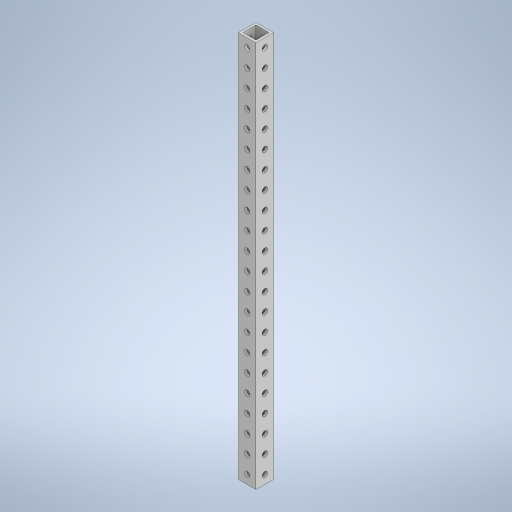
# Autodesk Inventor part: DriveHouseConnector-Length
Saved by Autodesk Inventor 2023 (Build 270158000, 158)
## iProperties
Created: 2022-09-20
Part Number: DriveHouseConnector-Length
Material: Generic
Document SubType Name: Modeling
Designer: seene
Density: 1 g/cm^3
Appearance: Default
Author: seene
Autodesk Inventor part; units mm, degrees
ref_plane "YZ Plane" through (0, 0, 0) normal (1, 0, 0) x (0, 1, 0)
ref_plane "XZ Plane" through (0, 0, 0) normal (0, 1, 0) x (-1, 0, 0)
ref_plane "XY Plane" through (0, 0, 0) normal (0, 0, 1) x (1, 0, 0)
sketch "Sketch1" plane through (0, 0, 0) normal (0, 1, 0) x (-1, 0, 0)
  line L0 (-12.7, 12.7) -> (12.7, 12.7)
  line L1 (12.7, 12.7) -> (12.7, -12.7)
  line L2 (12.7, -12.7) -> (-12.7, -12.7)
  line L3 (-12.7, -12.7) -> (-12.7, 12.7)
  line L4 (-12.7, 12.7) -> (12.7, -12.7) construction
  line L5 (12.7, 12.7) -> (-12.7, -12.7) construction
  line L6 (9.525, -9.525) -> (9.525, 9.525)
  line L7 (9.525, 9.525) -> (-9.525, 9.525)
  line L8 (-9.525, 9.525) -> (-9.525, -9.525)
  line L9 (-9.525, -9.525) -> (9.525, -9.525)
  point P0 (0, 0)
  dimension "d0" = 25.4
  dimension "d1" = 25.4
  dimension "d2" = 3.175
  constraints: 20 end point, 4 parallel, 2 midpoint, 2 perpendicular, 1 horizontal, 3 other
  measures "d0" distance of L1.end L2.end
  measures "d1" distance of L0.end L1.end
  measures "d2" distance between parallel lines of L1 L6
extrude "Extrusion1" add sketch "Sketch1" along normal blind 558.8
sketch "Sketch3" plane through (12.7, 0, 12.7) normal (1, 0, 0) x (0, 0, -1)
  line L0 (0, 0) -> (25.4, 0) projected
  line L1 (0, 0) -> (0, 558.8) projected
  point P0 (12.7, 0)
  point P1 (12.7, 12.7)
  dimension "d5" = 12.7
  dimension "d6" = 12.7
  measures "d5" distance from line of L0 point (12.7, 12.7)
  measures "d6" distance from line of L1 point (12.7, 12.7)
hole "Hole1" at (0, 12.7, 12.7) direction (0, 0, -1) diameter 7.9375 end through all
sketch "Sketch4" plane through (-12.7, 0, 12.7) normal (0, 0, 1) x (1, 0, 0)
  line L0 (0, 0) -> (25.4, 0) projected
  line L1 (25.4, 0) -> (25.4, 558.8) projected
  point P0 (12.7, 0)
  point P1 (12.7, 12.7)
  dimension "d8" = 12.7
  dimension "d10" = 12.7
  measures "d8" distance from line of L0 point (12.7, 12.7)
  measures "d10" distance from line of L1 point (12.7, 12.7)
hole "Hole2" at (12.7, 12.7, 0) direction (-1, 0, 0) diameter 7.9375 end through all
pattern_linear "Rectangular Pattern1" count 22 spacing 25.4 along (0, 1, 0) of "Hole1"
pattern_linear "Rectangular Pattern2" count 22 spacing 25.4 along (0, 1, 0) of "Hole2"
equation "\"d5\" = d10"
equation "\"d6\" = 0.5 * d0"
equation "\"d8\" = 0.5 * d0"
equation "\"d10\" = 0.5 * d0"
body "Solid1"
